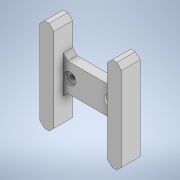
# Autodesk Inventor part: Fan_feet
Saved by Autodesk Inventor 2022 (Build 260153000, 153)
## iProperties
Created: 2022-04-11
Part Number: Fan_feet
Material: Generic
Document SubType Name: Modeling
Designer: Dani
Density: 1 g/cm^3
Appearance: Default
Author: Dani
## iProperties of the stored document Fan_feet_3DPrint.ipt
Created: 2022-04-11
Part Number: Fan_feet_3DPrint
Material: Generic
Document SubType Name: Modeling
Designer: Dani
Density: 1 g/cm^3
Appearance: Default
Author: Dani
Autodesk Inventor part; units mm, degrees
ref_plane "YZ Plane" through (0, 0, 0) normal (1, 0, 0) x (0, 1, 0)
ref_plane "XZ Plane" through (0, 0, 0) normal (0, 1, 0) x (-1, 0, 0)
ref_plane "XY Plane" through (0, 0, 0) normal (0, 0, 1) x (1, 0, 0)
sketch "Sketch1" plane through (0, 0, 0) normal (0, 0, 1) x (1, 0, 0)
  line L0 (0, 0) -> (70, 0)
  line L1 (70, 0) -> (70, 80)
  line L2 (70, 80) -> (0, 80)
  line L3 (0, 80) -> (0, 0)
  line L4 (12, 80) -> (58, 80)
  line L5 (58, 80) -> (58, 0)
  line L6 (58, 0) -> (12, 0)
  line L7 (12, 0) -> (12, 80)
  point P0 (18, 40)
  point P1 (52, 40)
  point P2 (12, 0)
  dimension "d0" = 70
  dimension "d1" = 80
  dimension "d2" = 34
  dimension "d3" = 18
  dimension "d6" = 40
  dimension "d7" = 40
  dimension "d8" = 12
  dimension "d9" = 12
  constraints: 16 end point, 4 parallel, 2 horizontal, 2 perpendicular, 2 point on line
  measures "d0" distance between parallel lines of L1 L3
  measures "d1" distance between parallel lines of L0 L2
  measures "d2" distance of point (52, 40) point (18, 40)
  measures "d3" distance from line of L3 point (18, 40)
  measures "d6" distance from line of L0 point (18, 40)
  measures "d7" distance from line of L0 point (52, 40)
  measures "d8" distance between parallel lines of L3 L7
  measures "d9" distance between parallel lines of L1 L5
extrude "Extrusion1" add sketch "Sketch1" against normal blind 6
extrude "Extrusion2" add sketch "Sketch1" along normal blind 10 contours L3 L2 L7 L0 | L5 L2 L1 L0
hole "Hole1" at (18, 40, 0) at (52, 40, 0) direction (0, 0, -1) diameter 4 depth 6
sketch "Sketch2" plane through (0, 0, 0) normal (0, 0, 1) x (1, 0, 0)
  line L0 (12, 0) -> (12, 80) projected
  line L1 (58, 0) -> (58, 80) projected
  line L2 (12, 0) -> (58, 0)
  line L3 (58, 0) -> (58, 28)
  line L4 (58, 28) -> (12, 28)
  line L5 (12, 28) -> (12, 0)
  line L6 (58, 80) -> (12, 80) projected
  line L7 (12, 80) -> (58, 80)
  line L8 (58, 80) -> (58, 52)
  line L9 (58, 52) -> (12, 52)
  line L10 (12, 52) -> (12, 80)
  point P0 (0, 0)
  point P1 (12, 52)
  dimension "d24" = 24
  dimension "d25" = 28
  constraints: 16 end point, 4 parallel, 2 horizontal, 2 perpendicular, 2 point on line
  measures "d24" distance between parallel lines of L9 L4
  measures "d25" distance between parallel lines of L6 L9
extrude "Extrusion3" cut sketch "Sketch2" against normal blind 6 contours L0 L4 L1 L2 | L0 L6 L1 L9
sketch "Sketch3" plane through (0, 0, 0) normal (0, 0, 1) x (1, 0, 0)
  line L0 (58, 28) -> (12, 28) projected
  line L1 (12, 52) -> (58, 52) projected
  line L2 (58, 28) -> (12, 28)
  line L3 (12, 28) -> (12, 52)
  line L4 (12, 52) -> (58, 52)
  line L5 (58, 52) -> (58, 28)
  circle A0 centre (52, 40) radius 2 projected
  circle A1 centre (52, 40) radius 5
  circle A2 centre (18, 40) radius 2 projected
  circle A3 centre (18, 40) radius 5
  point P0 (0, 0)
  dimension "d28" = 10
  dimension "d29" = 10
  constraints: 8 end point, 2 centre point, 2 coincident, 2 parallel, 1 horizontal, 1 perpendicular
  measures "d28" diameter of A1
  measures "d29" diameter of A3
extrude "Extrusion4" add sketch "Sketch3" along normal blind 2 contours L0 L3 L1 L5
chamfer "Chamfer2" distance 4 angle 45 12 edges at (58, 0, 2) (70, 0, 2) (12, 0, 2) (0, 0, 2) (70, 80, 2) (58, 80, 2) (12, 80, 2) (0, 80, 2) (58, 52, -2) (12, 52, -2) (58, 28, -2) (12, 28, -2)
body "Solid1"
